Autodesk Inventor part; units mm, degrees
(part 2 of 3)
  arc A350 (-686.435, 453.5902) -> (-694.055, 457.9897) centre (-691.515, 453.5902) ccw
  line L271 (-686.435, 453.5902) -> (-686.435, 424.2609)
  arc A351 (-694.055, 419.8614) -> (-686.435, 424.2609) centre (-691.515, 424.2609) ccw
  circle A352 centre (-532.765, 207.2233) radius 11.43 construction
  line L272 (-518.795, 211.6228) -> (-493.395, 226.2874)
  arc A353 (-485.775, 221.888) -> (-493.395, 226.2874) centre (-490.855, 221.888) ccw
  line L273 (-485.775, 221.888) -> (-485.775, 192.5586)
  arc A354 (-493.395, 188.1592) -> (-485.775, 192.5586) centre (-490.855, 192.5586) ccw
  line L274 (-493.395, 188.1592) -> (-518.795, 202.8239)
  arc A355 (-518.795, 211.6228) -> (-518.795, 202.8239) centre (-516.255, 207.2233) ccw
  line L275 (-529.59, 221.5214) -> (-529.59, 250.8508)
  arc A356 (-521.97, 255.2502) -> (-529.59, 250.8508) centre (-524.51, 250.8508) ccw
  line L276 (-521.97, 255.2502) -> (-496.57, 240.5855)
  arc A357 (-496.57, 231.7867) -> (-496.57, 240.5855) centre (-499.11, 236.1861) ccw
  line L277 (-496.57, 231.7867) -> (-521.97, 217.122)
  arc A358 (-529.59, 221.5214) -> (-521.97, 217.122) centre (-524.51, 221.5214) ccw
  line L278 (-543.56, 217.122) -> (-568.96, 231.7867)
  arc A359 (-568.96, 240.5855) -> (-568.96, 231.7867) centre (-566.42, 236.1861) ccw
  line L279 (-568.96, 240.5855) -> (-543.56, 255.2502)
  arc A360 (-535.94, 250.8508) -> (-543.56, 255.2502) centre (-541.02, 250.8508) ccw
  line L280 (-535.94, 250.8508) -> (-535.94, 221.5214)
  arc A361 (-543.56, 217.122) -> (-535.94, 221.5214) centre (-541.02, 221.5214) ccw
  line L281 (-546.735, 202.8239) -> (-572.135, 188.1592)
  arc A362 (-579.755, 192.5586) -> (-572.135, 188.1592) centre (-574.675, 192.5586) ccw
  line L282 (-579.755, 192.5586) -> (-579.755, 221.888)
  arc A363 (-572.135, 226.2874) -> (-579.755, 221.888) centre (-574.675, 221.888) ccw
  line L283 (-572.135, 226.2874) -> (-546.735, 211.6228)
  arc A364 (-546.735, 202.8239) -> (-546.735, 211.6228) centre (-549.275, 207.2233) ccw
  line L284 (-535.94, 192.9253) -> (-535.94, 163.5959)
  arc A365 (-543.56, 159.1965) -> (-535.94, 163.5959) centre (-541.02, 163.5959) ccw
  line L285 (-543.56, 159.1965) -> (-568.96, 173.8612)
  arc A366 (-568.96, 182.66) -> (-568.96, 173.8612) centre (-566.42, 178.2606) ccw
  line L286 (-568.96, 182.66) -> (-543.56, 197.3247)
  arc A367 (-535.94, 192.9253) -> (-543.56, 197.3247) centre (-541.02, 192.9253) ccw
  circle A368 centre (-532.765, 265.1489) radius 11.43 construction
  line L287 (-485.775, 279.8136) -> (-485.775, 250.4842)
  arc A369 (-485.775, 279.8136) -> (-493.395, 284.213) centre (-490.855, 279.8136) ccw
  arc A370 (-493.395, 246.0848) -> (-485.775, 250.4842) centre (-490.855, 250.4842) ccw
  line L288 (-493.395, 246.0848) -> (-518.795, 260.7495)
  arc A371 (-518.795, 269.5483) -> (-518.795, 260.7495) centre (-516.255, 265.1489) ccw
  line L289 (-518.795, 269.5483) -> (-493.395, 284.213)
  circle A372 centre (-532.765, 265.1489) radius 11.43 construction
  line L290 (-521.97, 313.1758) -> (-496.57, 298.5111)
  arc A373 (-521.97, 313.1758) -> (-529.59, 308.7764) centre (-524.51, 308.7764) ccw
  arc A374 (-496.57, 289.7123) -> (-496.57, 298.5111) centre (-499.11, 294.1117) ccw
  line L291 (-496.57, 289.7123) -> (-521.97, 275.0476)
  arc A375 (-529.59, 279.447) -> (-521.97, 275.0476) centre (-524.51, 279.447) ccw
  line L292 (-529.59, 279.447) -> (-529.59, 308.7764)
  circle A376 centre (-532.765, 265.1489) radius 11.43 construction
  line L293 (-568.96, 298.5111) -> (-543.56, 313.1758)
  arc A377 (-568.96, 298.5111) -> (-568.96, 289.7123) centre (-566.42, 294.1117) ccw
  arc A378 (-535.94, 308.7764) -> (-543.56, 313.1758) centre (-541.02, 308.7764) ccw
  line L294 (-535.94, 308.7764) -> (-535.94, 279.447)
  arc A379 (-543.56, 275.0476) -> (-535.94, 279.447) centre (-541.02, 279.447) ccw
  line L295 (-543.56, 275.0476) -> (-568.96, 289.7123)
  circle A380 centre (-532.765, 265.1489) radius 11.43 construction
  line L296 (-579.755, 250.4842) -> (-579.755, 279.8136)
  arc A381 (-579.755, 250.4842) -> (-572.135, 246.0848) centre (-574.675, 250.4842) ccw
  arc A382 (-572.135, 284.213) -> (-579.755, 279.8136) centre (-574.675, 279.8136) ccw
  line L297 (-572.135, 284.213) -> (-546.735, 269.5483)
  arc A383 (-546.735, 260.7495) -> (-546.735, 269.5483) centre (-549.275, 265.1489) ccw
  line L298 (-546.735, 260.7495) -> (-572.135, 246.0848)
  circle A384 centre (-532.765, 265.1489) radius 11.43 construction
  line L299 (-543.56, 217.122) -> (-568.96, 231.7867)
  arc A385 (-543.56, 217.122) -> (-535.94, 221.5214) centre (-541.02, 221.5214) ccw
  arc A386 (-568.96, 240.5855) -> (-568.96, 231.7867) centre (-566.42, 236.1861) ccw
  line L300 (-568.96, 240.5855) -> (-543.56, 255.2502)
  arc A387 (-535.94, 250.8508) -> (-543.56, 255.2502) centre (-541.02, 250.8508) ccw
  line L301 (-535.94, 250.8508) -> (-535.94, 221.5214)
  circle A388 centre (-532.765, 265.1489) radius 11.43 construction
  circle A389 centre (-582.93, 236.1861) radius 11.43 construction
  circle A390 centre (-633.095, 265.1489) radius 11.43 construction
  line L302 (-586.105, 279.8136) -> (-586.105, 250.4842)
  arc A391 (-593.725, 246.0848) -> (-586.105, 250.4842) centre (-591.185, 250.4842) ccw
  arc A392 (-619.125, 269.5483) -> (-619.125, 260.7495) centre (-616.585, 265.1489) ccw
  line L303 (-593.725, 246.0848) -> (-619.125, 260.7495)
  line L304 (-619.125, 269.5483) -> (-593.725, 284.213)
  arc A393 (-586.105, 279.8136) -> (-593.725, 284.213) centre (-591.185, 279.8136) ccw
  line L305 (-622.3, 313.1758) -> (-596.9, 298.5111)
  arc A394 (-596.9, 289.7123) -> (-596.9, 298.5111) centre (-599.44, 294.1117) ccw
  arc A395 (-629.92, 279.447) -> (-622.3, 275.0476) centre (-624.84, 279.447) ccw
  line L306 (-596.9, 289.7123) -> (-622.3, 275.0476)
  line L307 (-629.92, 279.447) -> (-629.92, 308.7764)
  arc A396 (-622.3, 313.1758) -> (-629.92, 308.7764) centre (-624.84, 308.7764) ccw
  line L308 (-669.29, 298.5111) -> (-643.89, 313.1758)
  arc A397 (-636.27, 308.7764) -> (-643.89, 313.1758) centre (-641.35, 308.7764) ccw
  arc A398 (-643.89, 275.0476) -> (-636.27, 279.447) centre (-641.35, 279.447) ccw
  line L309 (-636.27, 308.7764) -> (-636.27, 279.447)
  line L310 (-643.89, 275.0476) -> (-669.29, 289.7123)
  arc A399 (-669.29, 298.5111) -> (-669.29, 289.7123) centre (-666.75, 294.1117) ccw
  line L311 (-680.085, 250.4842) -> (-680.085, 279.8136)
  arc A400 (-672.465, 284.213) -> (-680.085, 279.8136) centre (-675.005, 279.8136) ccw
  arc A401 (-647.065, 260.7495) -> (-647.065, 269.5483) centre (-649.605, 265.1489) ccw
  line L312 (-672.465, 284.213) -> (-647.065, 269.5483)
  line L313 (-647.065, 260.7495) -> (-672.465, 246.0848)
  arc A402 (-680.085, 250.4842) -> (-672.465, 246.0848) centre (-675.005, 250.4842) ccw
  line L314 (-643.89, 217.122) -> (-669.29, 231.7867)
  arc A403 (-669.29, 240.5855) -> (-669.29, 231.7867) centre (-666.75, 236.1861) ccw
  arc A404 (-636.27, 250.8508) -> (-643.89, 255.2502) centre (-641.35, 250.8508) ccw
  line L315 (-669.29, 240.5855) -> (-643.89, 255.2502)
  line L316 (-636.27, 250.8508) -> (-636.27, 221.5214)
  arc A405 (-643.89, 217.122) -> (-636.27, 221.5214) centre (-641.35, 221.5214) ccw
  circle A406 centre (-582.93, 294.1117) radius 11.43 construction
  circle A407 centre (-633.095, 323.0744) radius 11.43 construction
  circle A408 centre (-482.6, 294.1117) radius 11.43 construction
  circle A409 centre (-482.6, 352.0372) radius 11.43 construction
  circle A410 centre (-532.765, 323.0744) radius 11.43 construction
  line L317 (-521.97, 313.1758) -> (-496.57, 298.5111)
  arc A411 (-496.57, 289.7123) -> (-496.57, 298.5111) centre (-499.11, 294.1117) ccw
  line L318 (-496.57, 289.7123) -> (-521.97, 275.0476)
  arc A412 (-529.59, 279.447) -> (-521.97, 275.0476) centre (-524.51, 279.447) ccw
  line L319 (-529.59, 279.447) -> (-529.59, 308.7764)
  arc A413 (-521.97, 313.1758) -> (-529.59, 308.7764) centre (-524.51, 308.7764) ccw
  line L320 (-518.795, 327.4739) -> (-493.395, 342.1386)
  arc A414 (-485.775, 337.7391) -> (-493.395, 342.1386) centre (-490.855, 337.7391) ccw
  line L321 (-485.775, 337.7391) -> (-485.775, 308.4098)
  arc A415 (-493.395, 304.0103) -> (-485.775, 308.4098) centre (-490.855, 308.4098) ccw
  line L322 (-493.395, 304.0103) -> (-518.795, 318.675)
  arc A416 (-518.795, 327.4739) -> (-518.795, 318.675) centre (-516.255, 323.0744) ccw
  line L323 (-529.59, 337.3725) -> (-529.59, 366.7019)
  arc A417 (-521.97, 371.1013) -> (-529.59, 366.7019) centre (-524.51, 366.7019) ccw
  line L324 (-521.97, 371.1013) -> (-496.57, 356.4366)
  arc A418 (-496.57, 347.6378) -> (-496.57, 356.4366) centre (-499.11, 352.0372) ccw
  line L325 (-496.57, 347.6378) -> (-521.97, 332.9731)
  arc A419 (-529.59, 337.3725) -> (-521.97, 332.9731) centre (-524.51, 337.3725) ccw
  line L326 (-543.56, 332.9731) -> (-568.96, 347.6378)
  arc A420 (-568.96, 356.4366) -> (-568.96, 347.6378) centre (-566.42, 352.0372) ccw
  line L327 (-568.96, 356.4366) -> (-543.56, 371.1013)
  arc A421 (-535.94, 366.7019) -> (-543.56, 371.1013) centre (-541.02, 366.7019) ccw
  line L328 (-535.94, 366.7019) -> (-535.94, 337.3725)
  arc A422 (-543.56, 332.9731) -> (-535.94, 337.3725) centre (-541.02, 337.3725) ccw
  line L329 (-546.735, 318.675) -> (-572.135, 304.0103)
  arc A423 (-579.755, 308.4098) -> (-572.135, 304.0103) centre (-574.675, 308.4098) ccw
  line L330 (-579.755, 308.4098) -> (-579.755, 337.7391)
  arc A424 (-572.135, 342.1386) -> (-579.755, 337.7391) centre (-574.675, 337.7391) ccw
  line L331 (-572.135, 342.1386) -> (-546.735, 327.4739)
  arc A425 (-546.735, 318.675) -> (-546.735, 327.4739) centre (-549.275, 323.0744) ccw
  line L332 (-586.105, 337.7391) -> (-586.105, 308.4098)
  arc A426 (-593.725, 304.0103) -> (-586.105, 308.4098) centre (-591.185, 308.4098) ccw
  line L333 (-593.725, 304.0103) -> (-619.125, 318.675)
  arc A427 (-619.125, 327.4739) -> (-619.125, 318.675) centre (-616.585, 323.0744) ccw
  line L334 (-619.125, 327.4739) -> (-593.725, 342.1386)
  arc A428 (-586.105, 337.7391) -> (-593.725, 342.1386) centre (-591.185, 337.7391) ccw
  line L335 (-622.3, 371.1013) -> (-596.9, 356.4366)
  arc A429 (-596.9, 347.6378) -> (-596.9, 356.4366) centre (-599.44, 352.0372) ccw
  line L336 (-596.9, 347.6378) -> (-622.3, 332.9731)
  arc A430 (-629.92, 337.3725) -> (-622.3, 332.9731) centre (-624.84, 337.3725) ccw
  line L337 (-629.92, 337.3725) -> (-629.92, 366.7019)
  arc A431 (-622.3, 371.1013) -> (-629.92, 366.7019) centre (-624.84, 366.7019) ccw
  line L338 (-669.29, 356.4366) -> (-643.89, 371.1013)
  arc A432 (-636.27, 366.7019) -> (-643.89, 371.1013) centre (-641.35, 366.7019) ccw
  line L339 (-636.27, 366.7019) -> (-636.27, 337.3725)
  arc A433 (-643.89, 332.9731) -> (-636.27, 337.3725) centre (-641.35, 337.3725) ccw
  line L340 (-643.89, 332.9731) -> (-669.29, 347.6378)
  arc A434 (-669.29, 356.4366) -> (-669.29, 347.6378) centre (-666.75, 352.0372) ccw
  line L341 (-680.085, 308.4098) -> (-680.085, 337.7391)
  arc A435 (-672.465, 342.1386) -> (-680.085, 337.7391) centre (-675.005, 337.7391) ccw
  line L342 (-672.465, 342.1386) -> (-647.065, 327.4739)
  arc A436 (-647.065, 318.675) -> (-647.065, 327.4739) centre (-649.605, 323.0744) ccw
  line L343 (-647.065, 318.675) -> (-672.465, 304.0103)
  arc A437 (-680.085, 308.4098) -> (-672.465, 304.0103) centre (-675.005, 308.4098) ccw
  line L344 (-643.89, 275.0476) -> (-669.29, 289.7123)
  arc A438 (-669.29, 298.5111) -> (-669.29, 289.7123) centre (-666.75, 294.1117) ccw
  line L345 (-669.29, 298.5111) -> (-643.89, 313.1758)
  arc A439 (-636.27, 308.7764) -> (-643.89, 313.1758) centre (-641.35, 308.7764) ccw
  line L346 (-636.27, 308.7764) -> (-636.27, 279.447)
  arc A440 (-643.89, 275.0476) -> (-636.27, 279.447) centre (-641.35, 279.447) ccw
  arc A441 (-485.775, 337.7391) -> (-493.395, 342.1386) centre (-490.855, 337.7391) ccw
  line L347 (-485.775, 337.7391) -> (-485.775, 308.4098)
  arc A442 (-493.395, 304.0103) -> (-485.775, 308.4098) centre (-490.855, 308.4098) ccw
  line L348 (-493.395, 304.0103) -> (-518.795, 318.675)
  arc A443 (-518.795, 327.4739) -> (-518.795, 318.675) centre (-516.255, 323.0744) ccw
  line L349 (-518.795, 327.4739) -> (-493.395, 342.1386)
  arc A444 (-471.805, 342.1386) -> (-479.425, 337.7391) centre (-474.345, 337.7391) ccw
  line L350 (-471.805, 342.1386) -> (-446.405, 327.4739)
  arc A445 (-446.405, 318.675) -> (-446.405, 327.4739) centre (-448.945, 323.0744) ccw
  line L351 (-446.405, 318.675) -> (-471.805, 304.0103)
  arc A446 (-479.425, 308.4098) -> (-471.805, 304.0103) centre (-474.345, 308.4098) ccw
  line L352 (-479.425, 308.4098) -> (-479.425, 337.7391)
  arc A447 (-468.63, 356.4366) -> (-468.63, 347.6378) centre (-466.09, 352.0372) ccw
  line L353 (-468.63, 356.4366) -> (-443.23, 371.1013)
  arc A448 (-435.61, 366.7019) -> (-443.23, 371.1013) centre (-440.69, 366.7019) ccw
  line L354 (-435.61, 366.7019) -> (-435.61, 337.3725)
  arc A449 (-443.23, 332.9731) -> (-435.61, 337.3725) centre (-440.69, 337.3725) ccw
  line L355 (-443.23, 332.9731) -> (-468.63, 347.6378)
  arc A450 (-479.425, 366.3353) -> (-471.805, 361.9359) centre (-474.345, 366.3353) ccw
  line L356 (-479.425, 366.3353) -> (-479.425, 395.6647)
  arc A451 (-471.805, 400.0641) -> (-479.425, 395.6647) centre (-474.345, 395.6647) ccw
  line L357 (-471.805, 400.0641) -> (-446.405, 385.3994)
  arc A452 (-446.405, 376.6006) -> (-446.405, 385.3994) centre (-448.945, 381) ccw
  line L358 (-446.405, 376.6006) -> (-471.805, 361.9359)
  arc A453 (-493.395, 361.9359) -> (-485.775, 366.3353) centre (-490.855, 366.3353) ccw
  line L359 (-493.395, 361.9359) -> (-518.795, 376.6006)
  arc A454 (-518.795, 385.3994) -> (-518.795, 376.6006) centre (-516.255, 381) ccw
  line L360 (-518.795, 385.3994) -> (-493.395, 400.0641)
  arc A455 (-485.775, 395.6647) -> (-493.395, 400.0641) centre (-490.855, 395.6647) ccw
  line L361 (-485.775, 395.6647) -> (-485.775, 366.3353)
  circle A456 centre (-532.765, 381) radius 11.43
  line L362 (-521.97, 371.1013) -> (-496.57, 356.4366)
  arc A457 (-496.57, 347.6378) -> (-496.57, 356.4366) centre (-499.11, 352.0372) ccw
  line L363 (-496.57, 347.6378) -> (-521.97, 332.9731)
  arc A458 (-529.59, 337.3725) -> (-521.97, 332.9731) centre (-524.51, 337.3725) ccw
  line L364 (-529.59, 337.3725) -> (-529.59, 366.7019)
  arc A459 (-521.97, 371.1013) -> (-529.59, 366.7019) centre (-524.51, 366.7019) ccw
  line L365 (-518.795, 385.3994) -> (-493.395, 400.0641)
  arc A460 (-485.775, 395.6647) -> (-493.395, 400.0641) centre (-490.855, 395.6647) ccw
  line L366 (-485.775, 395.6647) -> (-485.775, 366.3353)
  arc A461 (-493.395, 361.9359) -> (-485.775, 366.3353) centre (-490.855, 366.3353) ccw
  line L367 (-493.395, 361.9359) -> (-518.795, 376.6006)
  arc A462 (-518.795, 385.3994) -> (-518.795, 376.6006) centre (-516.255, 381) ccw
  line L368 (-529.59, 395.2981) -> (-529.59, 424.6275)
  arc A463 (-521.97, 429.0269) -> (-529.59, 424.6275) centre (-524.51, 424.6275) ccw
  line L369 (-521.97, 429.0269) -> (-496.57, 414.3622)
  arc A464 (-496.57, 405.5634) -> (-496.57, 414.3622) centre (-499.11, 409.9628) ccw
  line L370 (-496.57, 405.5634) -> (-521.97, 390.8987)
  arc A465 (-529.59, 395.2981) -> (-521.97, 390.8987) centre (-524.51, 395.2981) ccw
  line L371 (-543.56, 390.8987) -> (-568.96, 405.5634)
  arc A466 (-568.96, 414.3622) -> (-568.96, 405.5634) centre (-566.42, 409.9628) ccw
  line L372 (-568.96, 414.3622) -> (-543.56, 429.0269)
  arc A467 (-535.94, 424.6275) -> (-543.56, 429.0269) centre (-541.02, 424.6275) ccw
  line L373 (-535.94, 424.6275) -> (-535.94, 395.2981)
  arc A468 (-543.56, 390.8987) -> (-535.94, 395.2981) centre (-541.02, 395.2981) ccw
  line L374 (-546.735, 376.6006) -> (-572.135, 361.9359)
  arc A469 (-579.755, 366.3353) -> (-572.135, 361.9359) centre (-574.675, 366.3353) ccw
  line L375 (-579.755, 366.3353) -> (-579.755, 395.6647)
  arc A470 (-572.135, 400.0641) -> (-579.755, 395.6647) centre (-574.675, 395.6647) ccw
  line L376 (-572.135, 400.0641) -> (-546.735, 385.3994)
  arc A471 (-546.735, 376.6006) -> (-546.735, 385.3994) centre (-549.275, 381) ccw
  circle A472 centre (-582.93, 352.0372) radius 11.43
  line L377 (-586.105, 337.7391) -> (-586.105, 308.4098)
  arc A473 (-593.725, 304.0103) -> (-586.105, 308.4098) centre (-591.185, 308.4098) ccw
  line L378 (-593.725, 304.0103) -> (-619.125, 318.675)
  arc A474 (-619.125, 327.4739) -> (-619.125, 318.675) centre (-616.585, 323.0744) ccw
  line L379 (-619.125, 327.4739) -> (-593.725, 342.1386)
  arc A475 (-586.105, 337.7391) -> (-593.725, 342.1386) centre (-591.185, 337.7391) ccw
  line L380 (-572.135, 342.1386) -> (-546.735, 327.4739)
  arc A476 (-546.735, 318.675) -> (-546.735, 327.4739) centre (-549.275, 323.0744) ccw
  line L381 (-546.735, 318.675) -> (-572.135, 304.0103)
  arc A477 (-579.755, 308.4098) -> (-572.135, 304.0103) centre (-574.675, 308.4098) ccw
  line L382 (-579.755, 308.4098) -> (-579.755, 337.7391)
  arc A478 (-572.135, 342.1386) -> (-579.755, 337.7391) centre (-574.675, 337.7391) ccw
  line L383 (-568.96, 356.4366) -> (-543.56, 371.1013)
  arc A479 (-535.94, 366.7019) -> (-543.56, 371.1013) centre (-541.02, 366.7019) ccw
  line L384 (-535.94, 366.7019) -> (-535.94, 337.3725)
  arc A480 (-543.56, 332.9731) -> (-535.94, 337.3725) centre (-541.02, 337.3725) ccw
  line L385 (-543.56, 332.9731) -> (-568.96, 347.6378)
  arc A481 (-568.96, 356.4366) -> (-568.96, 347.6378) centre (-566.42, 352.0372) ccw
  line L386 (-579.755, 366.3353) -> (-579.755, 395.6647)
  arc A482 (-572.135, 400.0641) -> (-579.755, 395.6647) centre (-574.675, 395.6647) ccw
  line L387 (-572.135, 400.0641) -> (-546.735, 385.3994)
  arc A483 (-546.735, 376.6006) -> (-546.735, 385.3994) centre (-549.275, 381) ccw
  line L388 (-546.735, 376.6006) -> (-572.135, 361.9359)
  arc A484 (-579.755, 366.3353) -> (-572.135, 361.9359) centre (-574.675, 366.3353) ccw
  line L389 (-593.725, 361.9359) -> (-619.125, 376.6006)
  arc A485 (-619.125, 385.3994) -> (-619.125, 376.6006) centre (-616.585, 381) ccw
  line L390 (-619.125, 385.3994) -> (-593.725, 400.0641)
  arc A486 (-586.105, 395.6647) -> (-593.725, 400.0641) centre (-591.185, 395.6647) ccw
  line L391 (-586.105, 395.6647) -> (-586.105, 366.3353)
  arc A487 (-593.725, 361.9359) -> (-586.105, 366.3353) centre (-591.185, 366.3353) ccw
  circle A488 centre (-633.095, 381) radius 11.43
  line L392 (-596.9, 405.5634) -> (-622.3, 390.8987)
  arc A489 (-596.9, 405.5634) -> (-596.9, 414.3622) centre (-599.44, 409.9628) ccw
  line L393 (-622.3, 429.0269) -> (-596.9, 414.3622)
  arc A490 (-622.3, 429.0269) -> (-629.92, 424.6275) centre (-624.84, 424.6275) ccw
  line L394 (-629.92, 395.2981) -> (-629.92, 424.6275)
  arc A491 (-629.92, 395.2981) -> (-622.3, 390.8987) centre (-624.84, 395.2981) ccw
  line L395 (-636.27, 424.6275) -> (-636.27, 395.2981)
  arc A492 (-636.27, 424.6275) -> (-643.89, 429.0269) centre (-641.35, 424.6275) ccw
  line L396 (-669.29, 414.3622) -> (-643.89, 429.0269)
  arc A493 (-669.29, 414.3622) -> (-669.29, 405.5634) centre (-666.75, 409.9628) ccw
  line L397 (-643.89, 390.8987) -> (-669.29, 405.5634)
  arc A494 (-643.89, 390.8987) -> (-636.27, 395.2981) centre (-641.35, 395.2981) ccw
  line L398 (-672.465, 400.0641) -> (-647.065, 385.3994)
  arc A495 (-672.465, 400.0641) -> (-680.085, 395.6647) centre (-675.005, 395.6647) ccw
  line L399 (-680.085, 366.3353) -> (-680.085, 395.6647)
  arc A496 (-680.085, 366.3353) -> (-672.465, 361.9359) centre (-675.005, 366.3353) ccw
  line L400 (-647.065, 376.6006) -> (-672.465, 361.9359)
  arc A497 (-647.065, 376.6006) -> (-647.065, 385.3994) centre (-649.605, 381) ccw
  line L401 (-669.29, 356.4366) -> (-643.89, 371.1013)
  arc A498 (-669.29, 356.4366) -> (-669.29, 347.6378) centre (-666.75, 352.0372) ccw
  line L402 (-643.89, 332.9731) -> (-669.29, 347.6378)
  arc A499 (-643.89, 332.9731) -> (-636.27, 337.3725) centre (-641.35, 337.3725) ccw
  line L403 (-636.27, 366.7019) -> (-636.27, 337.3725)
  arc A500 (-636.27, 366.7019) -> (-643.89, 371.1013) centre (-641.35, 366.7019) ccw
  line L404 (-629.92, 337.3725) -> (-629.92, 366.7019)
  arc A501 (-629.92, 337.3725) -> (-622.3, 332.9731) centre (-624.84, 337.3725) ccw
  line L405 (-596.9, 347.6378) -> (-622.3, 332.9731)
  arc A502 (-596.9, 347.6378) -> (-596.9, 356.4366) centre (-599.44, 352.0372) ccw
  line L406 (-622.3, 371.1013) -> (-596.9, 356.4366)
  arc A503 (-622.3, 371.1013) -> (-629.92, 366.7019) centre (-624.84, 366.7019) ccw
  circle A504 centre (-582.93, 409.9628) radius 11.43
  line L407 (-586.105, 395.6647) -> (-586.105, 366.3353)
  line L408 (-593.725, 361.9359) -> (-619.125, 376.6006)
  arc A505 (-619.125, 385.3994) -> (-619.125, 376.6006) centre (-616.585, 381) ccw
  line L409 (-619.125, 385.3994) -> (-593.725, 400.0641)
  arc A506 (-586.105, 395.6647) -> (-593.725, 400.0641) centre (-591.185, 395.6647) ccw
  arc A507 (-593.725, 361.9359) -> (-586.105, 366.3353) centre (-591.185, 366.3353) ccw
  line L410 (-572.135, 400.0641) -> (-546.735, 385.3994)
  line L411 (-546.735, 376.6006) -> (-572.135, 361.9359)
  arc A508 (-579.755, 366.3353) -> (-572.135, 361.9359) centre (-574.675, 366.3353) ccw
  line L412 (-579.755, 366.3353) -> (-579.755, 395.6647)
  arc A509 (-572.135, 400.0641) -> (-579.755, 395.6647) centre (-574.675, 395.6647) ccw
  arc A510 (-546.735, 376.6006) -> (-546.735, 385.3994) centre (-549.275, 381) ccw
  line L413 (-568.96, 414.3622) -> (-543.56, 429.0269)
  line L414 (-535.94, 424.6275) -> (-535.94, 395.2981)
  arc A511 (-543.56, 390.8987) -> (-535.94, 395.2981) centre (-541.02, 395.2981) ccw
  line L415 (-543.56, 390.8987) -> (-568.96, 405.5634)
  arc A512 (-568.96, 414.3622) -> (-568.96, 405.5634) centre (-566.42, 409.9628) ccw
  arc A513 (-535.94, 424.6275) -> (-543.56, 429.0269) centre (-541.02, 424.6275) ccw
  line L416 (-579.755, 424.2609) -> (-579.755, 453.5902)
  line L417 (-572.135, 457.9897) -> (-546.735, 443.325)
  arc A514 (-546.735, 434.5261) -> (-546.735, 443.325) centre (-549.275, 438.9256) ccw
  line L418 (-546.735, 434.5261) -> (-572.135, 419.8614)
  arc A515 (-579.755, 424.2609) -> (-572.135, 419.8614) centre (-574.675, 424.2609) ccw
  arc A516 (-572.135, 457.9897) -> (-579.755, 453.5902) centre (-574.675, 453.5902) ccw
  line L419 (-593.725, 419.8614) -> (-619.125, 434.5261)
  line L420 (-619.125, 443.325) -> (-593.725, 457.9897)
  arc A517 (-586.105, 453.5902) -> (-593.725, 457.9897) centre (-591.185, 453.5902) ccw
  line L421 (-586.105, 453.5902) -> (-586.105, 424.2609)
  arc A518 (-593.725, 419.8614) -> (-586.105, 424.2609) centre (-591.185, 424.2609) ccw
  arc A519 (-619.125, 443.325) -> (-619.125, 434.5261) centre (-616.585, 438.9256) ccw
  circle A520 centre (-633.095, 438.9256) radius 11.43
  line L422 (-596.9, 463.4889) -> (-622.3, 448.8242)
  arc A521 (-596.9, 463.4889) -> (-596.9, 472.2877) centre (-599.44, 467.8883) ccw
  line L423 (-622.3, 486.9524) -> (-596.9, 472.2877)
  arc A522 (-622.3, 486.9524) -> (-629.92, 482.553) centre (-624.84, 482.553) ccw
  line L424 (-629.92, 453.2236) -> (-629.92, 482.553)
  arc A523 (-629.92, 453.2236) -> (-622.3, 448.8242) centre (-624.84, 453.2236) ccw
  line L425 (-636.27, 482.553) -> (-636.27, 453.2236)
  arc A524 (-636.27, 482.553) -> (-643.89, 486.9524) centre (-641.35, 482.553) ccw
  line L426 (-669.29, 472.2877) -> (-643.89, 486.9524)
  arc A525 (-669.29, 472.2877) -> (-669.29, 463.4889) centre (-666.75, 467.8883) ccw
  line L427 (-643.89, 448.8242) -> (-669.29, 463.4889)
  arc A526 (-643.89, 448.8242) -> (-636.27, 453.2236) centre (-641.35, 453.2236) ccw
  line L428 (-672.465, 457.9897) -> (-647.065, 443.325)
  arc A527 (-672.465, 457.9897) -> (-680.085, 453.5902) centre (-675.005, 453.5902) ccw
  line L429 (-680.085, 424.2609) -> (-680.085, 453.5902)
  arc A528 (-680.085, 424.2609) -> (-672.465, 419.8614) centre (-675.005, 424.2609) ccw
  line L430 (-647.065, 434.5261) -> (-672.465, 419.8614)
  arc A529 (-647.065, 434.5261) -> (-647.065, 443.325) centre (-649.605, 438.9256) ccw
  line L431 (-669.29, 414.3622) -> (-643.89, 429.0269)
  arc A530 (-669.29, 414.3622) -> (-669.29, 405.5634) centre (-666.75, 409.9628) ccw
  line L432 (-643.89, 390.8987) -> (-669.29, 405.5634)
  arc A531 (-643.89, 390.8987) -> (-636.27, 395.2981) centre (-641.35, 395.2981) ccw
  line L433 (-636.27, 424.6275) -> (-636.27, 395.2981)
  arc A532 (-636.27, 424.6275) -> (-643.89, 429.0269) centre (-641.35, 424.6275) ccw
  line L434 (-629.92, 395.2981) -> (-629.92, 424.6275)
  arc A533 (-629.92, 395.2981) -> (-622.3, 390.8987) centre (-624.84, 395.2981) ccw
  line L435 (-596.9, 405.5634) -> (-622.3, 390.8987)
  arc A534 (-596.9, 405.5634) -> (-596.9, 414.3622) centre (-599.44, 409.9628) ccw
  line L436 (-622.3, 429.0269) -> (-596.9, 414.3622)
  arc A535 (-622.3, 429.0269) -> (-629.92, 424.6275) centre (-624.84, 424.6275) ccw
  circle A536 centre (-482.6, 409.9628) radius 11.43
  circle A537 centre (-532.765, 438.9256) radius 11.43
  circle A538 centre (-582.93, 467.8883) radius 11.43
  circle A539 centre (-633.095, 496.8511) radius 11.43
  arc A540 (-493.395, 361.9359) -> (-485.775, 366.3353) centre (-490.855, 366.3353) ccw
  arc A541 (-518.795, 385.3994) -> (-518.795, 376.6006) centre (-516.255, 381) ccw
  line L437 (-493.395, 361.9359) -> (-518.795, 376.6006)
  line L438 (-518.795, 385.3994) -> (-493.395, 400.0641)
  arc A542 (-485.775, 395.6647) -> (-493.395, 400.0641) centre (-490.855, 395.6647) ccw
  line L439 (-485.775, 395.6647) -> (-485.775, 366.3353)
  arc A543 (-446.405, 376.6006) -> (-446.405, 385.3994) centre (-448.945, 381) ccw
  arc A544 (-479.425, 366.3353) -> (-471.805, 361.9359) centre (-474.345, 366.3353) ccw
  line L440 (-446.405, 376.6006) -> (-471.805, 361.9359)
  line L441 (-479.425, 366.3353) -> (-479.425, 395.6647)
  arc A545 (-471.805, 400.0641) -> (-479.425, 395.6647) centre (-474.345, 395.6647) ccw
  line L442 (-471.805, 400.0641) -> (-446.405, 385.3994)
  arc A546 (-435.61, 424.6275) -> (-443.23, 429.0269) centre (-440.69, 424.6275) ccw
  arc A547 (-443.23, 390.8987) -> (-435.61, 395.2981) centre (-440.69, 395.2981) ccw
  line L443 (-435.61, 424.6275) -> (-435.61, 395.2981)
  line L444 (-443.23, 390.8987) -> (-468.63, 405.5634)
  arc A548 (-468.63, 414.3622) -> (-468.63, 405.5634) centre (-466.09, 409.9628) ccw
  line L445 (-468.63, 414.3622) -> (-443.23, 429.0269)
  arc A549 (-471.805, 457.9897) -> (-479.425, 453.5902) centre (-474.345, 453.5902) ccw
  arc A550 (-446.405, 434.5261) -> (-446.405, 443.325) centre (-448.945, 438.9256) ccw
  line L446 (-471.805, 457.9897) -> (-446.405, 443.325)
  line L447 (-446.405, 434.5261) -> (-471.805, 419.8614)
  arc A551 (-479.425, 424.2609) -> (-471.805, 419.8614) centre (-474.345, 424.2609) ccw
  line L448 (-479.425, 424.2609) -> (-479.425, 453.5902)
  arc A552 (-518.795, 443.325) -> (-518.795, 434.5261) centre (-516.255, 438.9256) ccw
  arc A553 (-485.775, 453.5902) -> (-493.395, 457.9897) centre (-490.855, 453.5902) ccw
  line L449 (-518.795, 443.325) -> (-493.395, 457.9897)
  line L450 (-485.775, 453.5902) -> (-485.775, 424.2609)
  arc A554 (-493.395, 419.8614) -> (-485.775, 424.2609) centre (-490.855, 424.2609) ccw
  line L451 (-493.395, 419.8614) -> (-518.795, 434.5261)
  line L452 (-535.94, 424.6275) -> (-535.94, 395.2981)
  line L453 (-543.56, 390.8987) -> (-568.96, 405.5634)
  arc A555 (-543.56, 390.8987) -> (-535.94, 395.2981) centre (-541.02, 395.2981) ccw
  arc A556 (-568.96, 414.3622) -> (-568.96, 405.5634) centre (-566.42, 409.9628) ccw
  line L454 (-568.96, 414.3622) -> (-543.56, 429.0269)
  arc A557 (-535.94, 424.6275) -> (-543.56, 429.0269) centre (-541.02, 424.6275) ccw
  line L455 (-521.97, 429.0269) -> (-496.57, 414.3622)
  line L456 (-496.57, 405.5634) -> (-521.97, 390.8987)
  arc A558 (-496.57, 405.5634) -> (-496.57, 414.3622) centre (-499.11, 409.9628) ccw
  arc A559 (-529.59, 395.2981) -> (-521.97, 390.8987) centre (-524.51, 395.2981) ccw
  line L457 (-529.59, 395.2981) -> (-529.59, 424.6275)
  arc A560 (-521.97, 429.0269) -> (-529.59, 424.6275) centre (-524.51, 424.6275) ccw
  line L458 (-518.795, 443.325) -> (-493.395, 457.9897)
  line L459 (-485.775, 453.5902) -> (-485.775, 424.2609)
  arc A561 (-485.775, 453.5902) -> (-493.395, 457.9897) centre (-490.855, 453.5902) ccw
  arc A562 (-493.395, 419.8614) -> (-485.775, 424.2609) centre (-490.855, 424.2609) ccw
  line L460 (-493.395, 419.8614) -> (-518.795, 434.5261)
  arc A563 (-518.795, 443.325) -> (-518.795, 434.5261) centre (-516.255, 438.9256) ccw
  line L461 (-529.59, 453.2236) -> (-529.59, 482.553)
  line L462 (-521.97, 486.9524) -> (-496.57, 472.2877)
  arc A564 (-521.97, 486.9524) -> (-529.59, 482.553) centre (-524.51, 482.553) ccw
  arc A565 (-496.57, 463.4889) -> (-496.57, 472.2877) centre (-499.11, 467.8883) ccw
  line L463 (-496.57, 463.4889) -> (-521.97, 448.8242)
  arc A566 (-529.59, 453.2236) -> (-521.97, 448.8242) centre (-524.51, 453.2236) ccw
  line L464 (-543.56, 448.8242) -> (-568.96, 463.4889)
  line L465 (-568.96, 472.2877) -> (-543.56, 486.9524)
  arc A567 (-568.96, 472.2877) -> (-568.96, 463.4889) centre (-566.42, 467.8883) ccw
  arc A568 (-535.94, 482.553) -> (-543.56, 486.9524) centre (-541.02, 482.553) ccw
  line L466 (-535.94, 482.553) -> (-535.94, 453.2236)
  arc A569 (-543.56, 448.8242) -> (-535.94, 453.2236) centre (-541.02, 453.2236) ccw
  arc A570 (-586.105, 453.5902) -> (-593.725, 457.9897) centre (-591.185, 453.5902) ccw
  line L467 (-586.105, 453.5902) -> (-586.105, 424.2609)
  arc A571 (-593.725, 419.8614) -> (-586.105, 424.2609) centre (-591.185, 424.2609) ccw
  line L468 (-593.725, 419.8614) -> (-619.125, 434.5261)
  arc A572 (-619.125, 443.325) -> (-619.125, 434.5261) centre (-616.585, 438.9256) ccw
  line L469 (-619.125, 443.325) -> (-593.725, 457.9897)
  arc A573 (-572.135, 457.9897) -> (-579.755, 453.5902) centre (-574.675, 453.5902) ccw
  line L470 (-572.135, 457.9897) -> (-546.735, 443.325)
  arc A574 (-546.735, 434.5261) -> (-546.735, 443.325) centre (-549.275, 438.9256) ccw
  line L471 (-546.735, 434.5261) -> (-572.135, 419.8614)
  arc A575 (-579.755, 424.2609) -> (-572.135, 419.8614) centre (-574.675, 424.2609) ccw
  line L472 (-579.755, 424.2609) -> (-579.755, 453.5902)
  arc A576 (-568.96, 472.2877) -> (-568.96, 463.4889) centre (-566.42, 467.8883) ccw
  line L473 (-568.96, 472.2877) -> (-543.56, 486.9524)
  arc A577 (-535.94, 482.553) -> (-543.56, 486.9524) centre (-541.02, 482.553) ccw
  line L474 (-535.94, 482.553) -> (-535.94, 453.2236)
  arc A578 (-543.56, 448.8242) -> (-535.94, 453.2236) centre (-541.02, 453.2236) ccw
  line L475 (-543.56, 448.8242) -> (-568.96, 463.4889)
  arc A579 (-579.755, 482.1864) -> (-572.135, 477.787) centre (-574.675, 482.1864) ccw
  line L476 (-579.755, 482.1864) -> (-579.755, 511.5158)
  arc A580 (-572.135, 515.9152) -> (-579.755, 511.5158) centre (-574.675, 511.5158) ccw
  line L477 (-572.135, 515.9152) -> (-546.735, 501.2505)
  arc A581 (-546.735, 492.4517) -> (-546.735, 501.2505) centre (-549.275, 496.8511) ccw
  line L478 (-546.735, 492.4517) -> (-572.135, 477.787)
  arc A582 (-593.725, 477.787) -> (-586.105, 482.1864) centre (-591.185, 482.1864) ccw
  line L479 (-593.725, 477.787) -> (-619.125, 492.4517)
  arc A583 (-619.125, 501.2505) -> (-619.125, 492.4517) centre (-616.585, 496.8511) ccw
  line L480 (-619.125, 501.2505) -> (-593.725, 515.9152)
  arc A584 (-586.105, 511.5158) -> (-593.725, 515.9152) centre (-591.185, 511.5158) ccw
  line L481 (-586.105, 511.5158) -> (-586.105, 482.1864)
  line L482 (-596.9, 521.4145) -> (-622.3, 506.7498)
  arc A585 (-596.9, 521.4145) -> (-596.9, 530.2133) centre (-599.44, 525.8139) ccw
  line L483 (-622.3, 544.878) -> (-596.9, 530.2133)
  arc A586 (-622.3, 544.878) -> (-629.92, 540.4786) centre (-624.84, 540.4786) ccw
  line L484 (-629.92, 511.1492) -> (-629.92, 540.4786)
  arc A587 (-629.92, 511.1492) -> (-622.3, 506.7498) centre (-624.84, 511.1492) ccw
  line L485 (-636.27, 540.4786) -> (-636.27, 511.1492)
  arc A588 (-636.27, 540.4786) -> (-643.89, 544.878) centre (-641.35, 540.4786) ccw
  line L486 (-669.29, 530.2133) -> (-643.89, 544.878)
  arc A589 (-669.29, 530.2133) -> (-669.29, 521.4145) centre (-666.75, 525.8139) ccw
  line L487 (-643.89, 506.7498) -> (-669.29, 521.4145)
  arc A590 (-643.89, 506.7498) -> (-636.27, 511.1492) centre (-641.35, 511.1492) ccw
  line L488 (-672.465, 515.9152) -> (-647.065, 501.2505)
  arc A591 (-672.465, 515.9152) -> (-680.085, 511.5158) centre (-675.005, 511.5158) ccw
  line L489 (-680.085, 482.1864) -> (-680.085, 511.5158)
  arc A592 (-680.085, 482.1864) -> (-672.465, 477.787) centre (-675.005, 482.1864) ccw
  line L490 (-647.065, 492.4517) -> (-672.465, 477.787)
  arc A593 (-647.065, 492.4517) -> (-647.065, 501.2505) centre (-649.605, 496.8511) ccw
  line L491 (-669.29, 472.2877) -> (-643.89, 486.9524)
  arc A594 (-669.29, 472.2877) -> (-669.29, 463.4889) centre (-666.75, 467.8883) ccw
  line L492 (-643.89, 448.8242) -> (-669.29, 463.4889)
  arc A595 (-643.89, 448.8242) -> (-636.27, 453.2236) centre (-641.35, 453.2236) ccw
  line L493 (-636.27, 482.553) -> (-636.27, 453.2236)
  arc A596 (-636.27, 482.553) -> (-643.89, 486.9524) centre (-641.35, 482.553) ccw
  line L494 (-629.92, 453.2236) -> (-629.92, 482.553)
  arc A597 (-629.92, 453.2236) -> (-622.3, 448.8242) centre (-624.84, 453.2236) ccw
  line L495 (-596.9, 463.4889) -> (-622.3, 448.8242)
  arc A598 (-596.9, 463.4889) -> (-596.9, 472.2877) centre (-599.44, 467.8883) ccw
  line L496 (-622.3, 486.9524) -> (-596.9, 472.2877)
  arc A599 (-622.3, 486.9524) -> (-629.92, 482.553) centre (-624.84, 482.553) ccw
  circle A600 centre (-633.095, 554.7767) radius 11.43
  line L497 (-335.28, 366.7019) -> (-335.28, 337.3725)
  line L498 (-622.3, 544.878) -> (-596.9, 530.2133)
  arc A601 (-596.9, 521.4145) -> (-596.9, 530.2133) centre (-599.44, 525.8139) ccw
  line L499 (-596.9, 521.4145) -> (-622.3, 506.7498)
  arc A602 (-629.92, 511.1492) -> (-622.3, 506.7498) centre (-624.84, 511.1492) ccw
  line L500 (-629.92, 511.1492) -> (-629.92, 540.4786)
  arc A603 (-622.3, 544.878) -> (-629.92, 540.4786) centre (-624.84, 540.4786) ccw
  line L501 (-321.31, 718.6546) -> (-295.91, 703.9899)
  line L502 (-619.125, 559.1761) -> (-593.725, 573.8408)
  arc A604 (-586.105, 569.4414) -> (-593.725, 573.8408) centre (-591.185, 569.4414) ccw
  line L503 (-586.105, 569.4414) -> (-586.105, 540.112)
  arc A605 (-593.725, 535.7126) -> (-586.105, 540.112) centre (-591.185, 540.112) ccw
  line L504 (-593.725, 535.7126) -> (-619.125, 550.3772)
  arc A606 (-619.125, 559.1761) -> (-619.125, 550.3772) centre (-616.585, 554.7767) ccw
  line L505 (-619.125, 906.7294) -> (-593.725, 921.3941)
  line L506 (-629.92, 569.0747) -> (-629.92, 598.4041)
  arc A607 (-622.3, 602.8035) -> (-629.92, 598.4041) centre (-624.84, 598.4041) ccw
  line L507 (-622.3, 602.8035) -> (-596.9, 588.1388)
  arc A608 (-596.9, 579.34) -> (-596.9, 588.1388) centre (-599.44, 583.7394) ccw
  line L508 (-596.9, 579.34) -> (-622.3, 564.6753)
  arc A609 (-629.92, 569.0747) -> (-622.3, 564.6753) centre (-624.84, 569.0747) ccw
  line L509 (-680.085, 540.112) -> (-680.085, 569.4414)
  arc A610 (-672.465, 573.8408) -> (-680.085, 569.4414) centre (-675.005, 569.4414) ccw
  line L510 (-672.465, 573.8408) -> (-647.065, 559.1761)
  arc A611 (-647.065, 550.3772) -> (-647.065, 559.1761) centre (-649.605, 554.7767) ccw
  line L511 (-647.065, 550.3772) -> (-672.465, 535.7126)
  arc A612 (-680.085, 540.112) -> (-672.465, 535.7126) centre (-675.005, 540.112) ccw
  circle A613 centre (-582.93, 525.8139) radius 11.43
  circle A614 centre (-582.93, 583.7394) radius 11.43
  arc A615 (-596.9, 521.4145) -> (-596.9, 530.2133) centre (-599.44, 525.8139) ccw
  line L512 (-596.9, 521.4145) -> (-622.3, 506.7498)
  arc A616 (-629.92, 511.1492) -> (-622.3, 506.7498) centre (-624.84, 511.1492) ccw
  line L513 (-629.92, 511.1492) -> (-629.92, 540.4786)
  arc A617 (-622.3, 544.878) -> (-629.92, 540.4786) centre (-624.84, 540.4786) ccw
  line L514 (-622.3, 544.878) -> (-596.9, 530.2133)
  arc A618 (-586.105, 511.5158) -> (-593.725, 515.9152) centre (-591.185, 511.5158) ccw
  line L515 (-586.105, 511.5158) -> (-586.105, 482.1864)
  arc A619 (-593.725, 477.787) -> (-586.105, 482.1864) centre (-591.185, 482.1864) ccw
  line L516 (-593.725, 477.787) -> (-619.125, 492.4517)
  arc A620 (-619.125, 501.2505) -> (-619.125, 492.4517) centre (-616.585, 496.8511) ccw
  line L517 (-619.125, 501.2505) -> (-593.725, 515.9152)
  arc A621 (-572.135, 515.9152) -> (-579.755, 511.5158) centre (-574.675, 511.5158) ccw
  line L518 (-572.135, 515.9152) -> (-546.735, 501.2505)
  arc A622 (-546.735, 492.4517) -> (-546.735, 501.2505) centre (-549.275, 496.8511) ccw
  line L519 (-546.735, 492.4517) -> (-572.135, 477.787)
  arc A623 (-579.755, 482.1864) -> (-572.135, 477.787) centre (-574.675, 482.1864) ccw
  line L520 (-579.755, 482.1864) -> (-579.755, 511.5158)
  arc A624 (-568.96, 530.2133) -> (-568.96, 521.4145) centre (-566.42, 525.8139) ccw
  line L521 (-568.96, 530.2133) -> (-543.56, 544.878)
  arc A625 (-535.94, 540.4786) -> (-543.56, 544.878) centre (-541.02, 540.4786) ccw
  line L522 (-535.94, 540.4786) -> (-535.94, 511.1492)
  arc A626 (-543.56, 506.7498) -> (-535.94, 511.1492) centre (-541.02, 511.1492) ccw
  line L523 (-543.56, 506.7498) -> (-568.96, 521.4145)
  arc A627 (-579.755, 540.112) -> (-572.135, 535.7126) centre (-574.675, 540.112) ccw
  line L524 (-579.755, 540.112) -> (-579.755, 569.4414)
  arc A628 (-572.135, 573.8408) -> (-579.755, 569.4414) centre (-574.675, 569.4414) ccw
  line L525 (-572.135, 573.8408) -> (-546.735, 559.1761)
  arc A629 (-546.735, 550.3772) -> (-546.735, 559.1761) centre (-549.275, 554.7767) ccw
  line L526 (-546.735, 550.3772) -> (-572.135, 535.7126)
  line L527 (-586.105, 569.4414) -> (-586.105, 540.112)
  line L528 (-593.725, 535.7126) -> (-619.125, 550.3772)
  arc A630 (-593.725, 535.7126) -> (-586.105, 540.112) centre (-591.185, 540.112) ccw
  arc A631 (-619.125, 559.1761) -> (-619.125, 550.3772) centre (-616.585, 554.7767) ccw
  line L529 (-619.125, 559.1761) -> (-593.725, 573.8408)
  arc A632 (-586.105, 569.4414) -> (-593.725, 573.8408) centre (-591.185, 569.4414) ccw
  line L530 (-572.135, 573.8408) -> (-546.735, 559.1761)
  line L531 (-546.735, 550.3772) -> (-572.135, 535.7126)
  arc A633 (-546.735, 550.3772) -> (-546.735, 559.1761) centre (-549.275, 554.7767) ccw
  arc A634 (-579.755, 540.112) -> (-572.135, 535.7126) centre (-574.675, 540.112) ccw
  line L532 (-579.755, 540.112) -> (-579.755, 569.4414)
  arc A635 (-572.135, 573.8408) -> (-579.755, 569.4414) centre (-574.675, 569.4414) ccw
  line L533 (-568.96, 588.1388) -> (-543.56, 602.8035)
  line L534 (-535.94, 598.4041) -> (-535.94, 569.0747)
  arc A636 (-535.94, 598.4041) -> (-543.56, 602.8035) centre (-541.02, 598.4041) ccw
  arc A637 (-543.56, 564.6753) -> (-535.94, 569.0747) centre (-541.02, 569.0747) ccw
  line L535 (-543.56, 564.6753) -> (-568.96, 579.34)
  arc A638 (-568.96, 588.1388) -> (-568.96, 579.34) centre (-566.42, 583.7394) ccw
  line L536 (-579.755, 598.0375) -> (-579.755, 627.3669)
  line L537 (-572.135, 631.7663) -> (-546.735, 617.1016)
  arc A639 (-572.135, 631.7663) -> (-579.755, 627.3669) centre (-574.675, 627.3669) ccw
  arc A640 (-546.735, 608.3028) -> (-546.735, 617.1016) centre (-549.275, 612.7022) ccw
  line L538 (-546.735, 608.3028) -> (-572.135, 593.6381)
  arc A641 (-579.755, 598.0375) -> (-572.135, 593.6381) centre (-574.675, 598.0375) ccw
  line L539 (-593.725, 593.6381) -> (-619.125, 608.3028)
  line L540 (-619.125, 617.1016) -> (-593.725, 631.7663)
  arc A642 (-619.125, 617.1016) -> (-619.125, 608.3028) centre (-616.585, 612.7022) ccw
  arc A643 (-586.105, 627.3669) -> (-593.725, 631.7663) centre (-591.185, 627.3669) ccw
  line L541 (-586.105, 627.3669) -> (-586.105, 598.0375)
  arc A644 (-593.725, 593.6381) -> (-586.105, 598.0375) centre (-591.185, 598.0375) ccw
  circle A645 centre (-532.765, 554.7767) radius 11.43
  circle A646 centre (-532.765, 496.8511) radius 11.43
  circle A647 centre (-482.6, 467.8883) radius 11.43
  circle A648 centre (-432.435, 438.9256) radius 11.43
  circle A649 centre (-532.765, 612.7022) radius 11.43
  line L542 (-418.465, 443.325) -> (-393.065, 457.9897)
  line L543 (-385.445, 453.5902) -> (-385.445, 424.2609)
  arc A650 (-393.065, 419.8614) -> (-385.445, 424.2609) centre (-390.525, 424.2609) ccw
  line L544 (-393.065, 419.8614) -> (-418.465, 434.5261)
  arc A651 (-385.445, 453.5902) -> (-393.065, 457.9897) centre (-390.525, 453.5902) ccw
  arc A652 (-418.465, 443.325) -> (-418.465, 434.5261) centre (-415.925, 438.9256) ccw
  line L545 (-429.26, 453.2236) -> (-429.26, 482.553)
  line L546 (-421.64, 486.9524) -> (-396.24, 472.2877)
  arc A653 (-396.24, 463.4889) -> (-396.24, 472.2877) centre (-398.78, 467.8883) ccw
  line L547 (-396.24, 463.4889) -> (-421.64, 448.8242)
  arc A654 (-421.64, 486.9524) -> (-429.26, 482.553) centre (-424.18, 482.553) ccw
  arc A655 (-429.26, 453.2236) -> (-421.64, 448.8242) centre (-424.18, 453.2236) ccw
  line L548 (-443.23, 448.8242) -> (-468.63, 463.4889)
  line L549 (-468.63, 472.2877) -> (-443.23, 486.9524)
  arc A656 (-435.61, 482.553) -> (-443.23, 486.9524) centre (-440.69, 482.553) ccw
  line L550 (-435.61, 482.553) -> (-435.61, 453.2236)
  arc A657 (-468.63, 472.2877) -> (-468.63, 463.4889) centre (-466.09, 467.8883) ccw
  arc A658 (-443.23, 448.8242) -> (-435.61, 453.2236) centre (-440.69, 453.2236) ccw
  line L551 (-446.405, 434.5261) -> (-471.805, 419.8614)
  line L552 (-479.425, 424.2609) -> (-479.425, 453.5902)
  arc A659 (-471.805, 457.9897) -> (-479.425, 453.5902) centre (-474.345, 453.5902) ccw
  line L553 (-471.805, 457.9897) -> (-446.405, 443.325)
  arc A660 (-479.425, 424.2609) -> (-471.805, 419.8614) centre (-474.345, 424.2609) ccw
  arc A661 (-446.405, 434.5261) -> (-446.405, 443.325) centre (-448.945, 438.9256) ccw
  line L554 (-435.61, 424.6275) -> (-435.61, 395.2981)
  line L555 (-443.23, 390.8987) -> (-468.63, 405.5634)
  arc A662 (-468.63, 414.3622) -> (-468.63, 405.5634) centre (-466.09, 409.9628) ccw
  line L556 (-468.63, 414.3622) -> (-443.23, 429.0269)
  arc A663 (-443.23, 390.8987) -> (-435.61, 395.2981) centre (-440.69, 395.2981) ccw
  arc A664 (-435.61, 424.6275) -> (-443.23, 429.0269) centre (-440.69, 424.6275) ccw
  line L557 (-485.775, 453.5902) -> (-485.775, 424.2609)
  arc A665 (-485.775, 453.5902) -> (-493.395, 457.9897) centre (-490.855, 453.5902) ccw
  line L558 (-518.795, 443.325) -> (-493.395, 457.9897)
  arc A666 (-518.795, 443.325) -> (-518.795, 434.5261) centre (-516.255, 438.9256) ccw
  line L559 (-493.395, 419.8614) -> (-518.795, 434.5261)
  arc A667 (-493.395, 419.8614) -> (-485.775, 424.2609) centre (-490.855, 424.2609) ccw
  line L560 (-471.805, 457.9897) -> (-446.405, 443.325)
  arc A668 (-471.805, 457.9897) -> (-479.425, 453.5902) centre (-474.345, 453.5902) ccw
  line L561 (-479.425, 424.2609) -> (-479.425, 453.5902)
  arc A669 (-479.425, 424.2609) -> (-471.805, 419.8614) centre (-474.345, 424.2609) ccw
  line L562 (-446.405, 434.5261) -> (-471.805, 419.8614)
  arc A670 (-446.405, 434.5261) -> (-446.405, 443.325) centre (-448.945, 438.9256) ccw
  line L563 (-468.63, 472.2877) -> (-443.23, 486.9524)
  arc A671 (-468.63, 472.2877) -> (-468.63, 463.4889) centre (-466.09, 467.8883) ccw
  line L564 (-443.23, 448.8242) -> (-468.63, 463.4889)
  arc A672 (-443.23, 448.8242) -> (-435.61, 453.2236) centre (-440.69, 453.2236) ccw
  line L565 (-435.61, 482.553) -> (-435.61, 453.2236)
  arc A673 (-435.61, 482.553) -> (-443.23, 486.9524) centre (-440.69, 482.553) ccw
  line L566 (-479.425, 482.1864) -> (-479.425, 511.5158)
  arc A674 (-479.425, 482.1864) -> (-471.805, 477.787) centre (-474.345, 482.1864) ccw
  line L567 (-446.405, 492.4517) -> (-471.805, 477.787)
  arc A675 (-446.405, 492.4517) -> (-446.405, 501.2505) centre (-448.945, 496.8511) ccw
  line L568 (-471.805, 515.9152) -> (-446.405, 501.2505)
  arc A676 (-471.805, 515.9152) -> (-479.425, 511.5158) centre (-474.345, 511.5158) ccw
  line L569 (-493.395, 477.787) -> (-518.795, 492.4517)
  arc A677 (-493.395, 477.787) -> (-485.775, 482.1864) centre (-490.855, 482.1864) ccw
  line L570 (-485.775, 511.5158) -> (-485.775, 482.1864)
  arc A678 (-485.775, 511.5158) -> (-493.395, 515.9152) centre (-490.855, 511.5158) ccw
  line L571 (-518.795, 501.2505) -> (-493.395, 515.9152)
  arc A679 (-518.795, 501.2505) -> (-518.795, 492.4517) centre (-516.255, 496.8511) ccw
  line L572 (-521.97, 544.878) -> (-496.57, 530.2133)
  arc A680 (-496.57, 521.4145) -> (-496.57, 530.2133) centre (-499.11, 525.8139) ccw
  line L573 (-496.57, 521.4145) -> (-521.97, 506.7498)
  arc A681 (-529.59, 511.1492) -> (-521.97, 506.7498) centre (-524.51, 511.1492) ccw
  line L574 (-529.59, 511.1492) -> (-529.59, 540.4786)
  arc A682 (-521.97, 544.878) -> (-529.59, 540.4786) centre (-524.51, 540.4786) ccw
  line L575 (-518.795, 559.1761) -> (-493.395, 573.8408)
  arc A683 (-485.775, 569.4414) -> (-493.395, 573.8408) centre (-490.855, 569.4414) ccw
  line L576 (-485.775, 569.4414) -> (-485.775, 540.112)
  arc A684 (-493.395, 535.7126) -> (-485.775, 540.112) centre (-490.855, 540.112) ccw
  line L577 (-493.395, 535.7126) -> (-518.795, 550.3772)
  arc A685 (-518.795, 559.1761) -> (-518.795, 550.3772) centre (-516.255, 554.7767) ccw
  line L578 (-529.59, 569.0747) -> (-529.59, 598.4041)
  arc A686 (-521.97, 602.8035) -> (-529.59, 598.4041) centre (-524.51, 598.4041) ccw
  line L579 (-521.97, 602.8035) -> (-496.57, 588.1388)
  arc A687 (-496.57, 579.34) -> (-496.57, 588.1388) centre (-499.11, 583.7394) ccw
  line L580 (-496.57, 579.34) -> (-521.97, 564.6753)
  arc A688 (-529.59, 569.0747) -> (-521.97, 564.6753) centre (-524.51, 569.0747) ccw
  line L581 (-543.56, 564.6753) -> (-568.96, 579.34)
  arc A689 (-568.96, 588.1388) -> (-568.96, 579.34) centre (-566.42, 583.7394) ccw
  line L582 (-568.96, 588.1388) -> (-543.56, 602.8035)
  arc A690 (-535.94, 598.4041) -> (-543.56, 602.8035) centre (-541.02, 598.4041) ccw
  line L583 (-535.94, 598.4041) -> (-535.94, 569.0747)
  arc A691 (-543.56, 564.6753) -> (-535.94, 569.0747) centre (-541.02, 569.0747) ccw
  line L584 (-546.735, 550.3772) -> (-572.135, 535.7126)
  arc A692 (-579.755, 540.112) -> (-572.135, 535.7126) centre (-574.675, 540.112) ccw
  line L585 (-579.755, 540.112) -> (-579.755, 569.4414)
  arc A693 (-572.135, 573.8408) -> (-579.755, 569.4414) centre (-574.675, 569.4414) ccw
  line L586 (-572.135, 573.8408) -> (-546.735, 559.1761)
  arc A694 (-546.735, 550.3772) -> (-546.735, 559.1761) centre (-549.275, 554.7767) ccw
  line L587 (-485.775, 627.3669) -> (-485.775, 598.0375)
  arc A695 (-493.395, 593.6381) -> (-485.775, 598.0375) centre (-490.855, 598.0375) ccw
  line L588 (-493.395, 593.6381) -> (-518.795, 608.3028)
  arc A696 (-518.795, 617.1016) -> (-518.795, 608.3028) centre (-516.255, 612.7022) ccw
  line L589 (-518.795, 617.1016) -> (-493.395, 631.7663)
  arc A697 (-485.775, 627.3669) -> (-493.395, 631.7663) centre (-490.855, 627.3669) ccw
  line L590 (-521.97, 660.7291) -> (-496.57, 646.0644)
  arc A698 (-496.57, 637.2656) -> (-496.57, 646.0644) centre (-499.11, 641.665) ccw
  line L591 (-496.57, 637.2656) -> (-521.97, 622.6009)
  arc A699 (-529.59, 627.0003) -> (-521.97, 622.6009) centre (-524.51, 627.0003) ccw
  line L592 (-529.59, 627.0003) -> (-529.59, 656.3297)
  arc A700 (-521.97, 660.7291) -> (-529.59, 656.3297) centre (-524.51, 656.3297) ccw
  line L593 (-568.96, 646.0644) -> (-543.56, 660.7291)
  arc A701 (-535.94, 656.3297) -> (-543.56, 660.7291) centre (-541.02, 656.3297) ccw
  line L594 (-535.94, 656.3297) -> (-535.94, 627.0003)
  arc A702 (-543.56, 622.6009) -> (-535.94, 627.0003) centre (-541.02, 627.0003) ccw
  line L595 (-543.56, 622.6009) -> (-568.96, 637.2656)
  arc A703 (-568.96, 646.0644) -> (-568.96, 637.2656) centre (-566.42, 641.665) ccw
  line L596 (-579.755, 598.0375) -> (-579.755, 627.3669)
  arc A704 (-572.135, 631.7663) -> (-579.755, 627.3669) centre (-574.675, 627.3669) ccw
  line L597 (-572.135, 631.7663) -> (-546.735, 617.1016)
  arc A705 (-546.735, 608.3028) -> (-546.735, 617.1016) centre (-549.275, 612.7022) ccw
  line L598 (-546.735, 608.3028) -> (-572.135, 593.6381)
  arc A706 (-579.755, 598.0375) -> (-572.135, 593.6381) centre (-574.675, 598.0375) ccw
  line L599 (-543.56, 564.6753) -> (-568.96, 579.34)
  arc A707 (-568.96, 588.1388) -> (-568.96, 579.34) centre (-566.42, 583.7394) ccw
  line L600 (-568.96, 588.1388) -> (-543.56, 602.8035)
  arc A708 (-535.94, 598.4041) -> (-543.56, 602.8035) centre (-541.02, 598.4041) ccw
  line L601 (-535.94, 598.4041) -> (-535.94, 569.0747)
  arc A709 (-543.56, 564.6753) -> (-535.94, 569.0747) centre (-541.02, 569.0747) ccw
  circle A710 centre (-432.435, 496.8511) radius 11.43
  circle A711 centre (-482.6, 525.8139) radius 11.43
  circle A712 centre (-482.6, 583.7394) radius 11.43
  circle A713 centre (-482.6, 641.665) radius 11.43
  line L602 (-485.775, 627.3669) -> (-485.775, 598.0375)
  arc A714 (-493.395, 593.6381) -> (-485.775, 598.0375) centre (-490.855, 598.0375) ccw
  line L603 (-493.395, 593.6381) -> (-518.795, 608.3028)
  arc A715 (-518.795, 617.1016) -> (-518.795, 608.3028) centre (-516.255, 612.7022) ccw
  line L604 (-518.795, 617.1016) -> (-493.395, 631.7663)
  arc A716 (-485.775, 627.3669) -> (-493.395, 631.7663) centre (-490.855, 627.3669) ccw
  line L605 (-471.805, 631.7663) -> (-446.405, 617.1016)
  arc A717 (-446.405, 608.3028) -> (-446.405, 617.1016) centre (-448.945, 612.7022) ccw
  line L606 (-446.405, 608.3028) -> (-471.805, 593.6381)
  arc A718 (-479.425, 598.0375) -> (-471.805, 593.6381) centre (-474.345, 598.0375) ccw
  line L607 (-479.425, 598.0375) -> (-479.425, 627.3669)
  arc A719 (-471.805, 631.7663) -> (-479.425, 627.3669) centre (-474.345, 627.3669) ccw
  line L608 (-468.63, 646.0644) -> (-443.23, 660.7291)
  arc A720 (-435.61, 656.3297) -> (-443.23, 660.7291) centre (-440.69, 656.3297) ccw
  line L609 (-435.61, 656.3297) -> (-435.61, 627.0003)
  arc A721 (-443.23, 622.6009) -> (-435.61, 627.0003) centre (-440.69, 627.0003) ccw